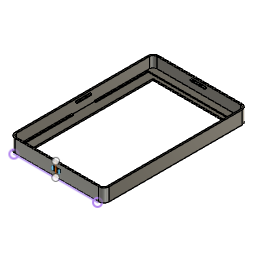
Front+Cover_small (Autodesk Fusion 360 archive; units mm, degrees)
design "Front Cover_small"
Autodesk Fusion 360 part; units mm, degrees
sketch "Outer Dimensions" plane through (0, 0, 0) normal (0, 0, 1) x (1, 0, 0)
  line L0 (117.36, 12) -> (117.36, 183)
  line L1 (125.5, 8.5) -> (125.5, 186.5)
  line L2 (16.04, 178.6) -> (16.04, 16.4)
  line L3 (112.96, 16.4) -> (112.96, 178.6)
  line L4 (3.5, 191.5) -> (125.5, 3.5) construction
  circle A0 centre (8.25, 8.75) radius 1.5
  line L5 (5.36, 12) -> (117.36, 12)
  circle A1 centre (120.75, 8.75) radius 1.5
  circle A2 centre (120.75, 186.25) radius 1.5
  line L6 (8.5, 3.5) -> (120.5, 3.5)
  line L7 (112.96, 178.6) -> (16.04, 16.4) construction
  line L8 (5.36, 82.4713) -> (1.5, 82.4713)
  line L9 (117.36, 183) -> (5.36, 183)
  line L10 (16.04, 16.4) -> (112.96, 16.4)
  line L11 (16.04, 178.6) -> (112.96, 16.4) construction
  line L12 (1.5, 112.5) -> (5.36, 112.5)
  circle A3 centre (8.25, 186.25) radius 1.5
  line L13 (120.5, 191.5) -> (8.5, 191.5)
  line L14 (5.36, 112.5) -> (5.36, 82.4713)
  line L15 (125.5, 191.5) -> (3.5, 3.5) construction
  line L16 (112.96, 178.6) -> (16.04, 178.6)
  line L17 (5.36, 183) -> (5.36, 12)
  line L18 (3.5, 186.5) -> (3.5, 8.5)
  arc A4 (8.5, 191.5) -> (3.5, 186.5) centre (8.5, 186.5) ccw
  arc A5 (3.5, 8.5) -> (8.5, 3.5) centre (8.5, 8.5) ccw
  arc A6 (120.5, 3.5) -> (125.5, 8.5) centre (120.5, 8.5) ccw
  arc A7 (125.5, 186.5) -> (120.5, 191.5) centre (120.5, 186.5) ccw
  line L19 (1.5, 186.5) -> (1.5, 8.5)
  arc A8 (1.5, 8.5) -> (8.5, 1.5) centre (8.5, 8.5) ccw
  line L20 (8.5, 1.5) -> (120.5, 1.5)
  arc A9 (120.5, 1.5) -> (127.5, 8.5) centre (120.5, 8.5) ccw
  line L21 (127.5, 8.5) -> (127.5, 186.5)
  arc A10 (127.5, 186.5) -> (120.5, 193.5) centre (120.5, 186.5) ccw
  line L22 (120.5, 193.5) -> (8.5, 193.5)
  arc A11 (8.5, 193.5) -> (1.5, 186.5) centre (8.5, 186.5) ccw
  point P0 (64.5, 97.5)
  point P1 (8.25, 186.25)
  point P2 (120.75, 8.75)
  point P3 (8.25, 8.75)
  point P4 (120.75, 186.25)
  point P5 (8.25, 8.75)
  point P6 (120.75, 8.75)
  point P7 (64.5, 97.5)
  point P8 (64.5, 97.5)
  point P9 (64.5, 97.5)
  point P10 (64.5, 97.5)
  dimension "d61" = 96.92
  dimension "d62" = 162.2
  dimension "d63" = 112
  dimension "d64" = 171
  dimension "d65" = 4.4
  dimension "d66" = 4.4
  dimension "d84" = 5
  dimension "d88" = 5
  dimension "d90" = 5
  dimension "d98" = 3
  dimension "d102" = 5.25
  dimension "d103" = 4.75
  dimension "d104" = 2
  dimension "d105" = 7
  dimension "d109" = 122
  dimension "d110" = 188
  constraint horizontal L16
  constraint perpendicular L2 L16
  constraint parallel L10 L16
  constraint parallel L2 L3
  constraint coincident P10 L7
  constraint coincident P10 L11
  constraint coincident P10 P9
  constraint horizontal L5
  constraint vertical L0
  constraint horizontal L9
  constraint vertical L17
  constraint horizontal L8
  constraint horizontal L12
  constraint vertical L14
  constraint coincident L8.start L17
  constraint coincident L4.start L18
  constraint coincident L4.start L13
  constraint tangent L18 A4
  constraint tangent L13 A4
  constraint coincident L15.start L13
  constraint coincident L15.start L1
  constraint coincident L15.end L18
  constraint coincident L15.end L6
  constraint tangent L18 A5
  constraint tangent L6 A5
  constraint coincident L4.end L6
  constraint coincident L4.end L1
  constraint tangent L6 A6
  constraint tangent L1 A6
  measures "d61" distance of L2.end L3.start
  measures "d62" distance of L2.start L2.end
  measures "d63" distance of L5.start L0.start
  measures "d64" distance of L9.end L5.start
  measures "d65" distance of L9 L16
  measures "d66" distance of L0 L3
  measures "d84" radius of A4
  measures "d88" radius of A5
  measures "d90" radius of A6
  measures "d98" diameter of A2
  measures "d102" distance of P4 L13
  measures "d103" distance of P4 L1
  measures "d105" radius of A10
  measures "d109" distance of L1 L18
  measures "d110" distance of L6 L13
extrude "Extrude7" add sketch "Outer Dimensions" along normal blind 2 contours L0 L5 L9 L14 L17 | L2 L3 L10 L16 makes body 1
extrude "Extrude9" add sketch "Outer Dimensions" along normal blind 2 contours L8 L12 L14 L17 L18 bodies 1
extrude "Extrude10" add sketch "Outer Dimensions" along normal blind 17.5 contours L1 L6 L8 L12 L13 L18 A4 A5 A6 A7 L19 A8 L20 A9 L21 A10 L22 A11 | L8 L12 L18 L19 bodies 1
extrude "Extrude11" add sketch "Outer Dimensions" along normal blind 3.2 separate body contours A0 | A1 | A2 | A3 makes body 2 at (121.1563, 187.6939, 2.1333) makes body 3 at (9.7425, 8.6006, 2.1333) makes body 4 at (9.0638, 184.99, 2.1333) makes body 5 at (120.2723, 7.3281, 2.1333)
extrude "Extrude14" add sketch "Outer Dimensions" along normal blind 3.2 contours L0 L1 L5 L6 L8 L9 L12 L13 L17 L18 A4 A5 A6 A7 bodies 1 2 3 4 5
extrude "Extrude12" cut sketch "Outer Dimensions" along normal blind 2 contours L2 L3 L10 L16 bodies 1
sketch "Sketch4" plane through (0, 0, 0) normal (0, 1, 0) x (1, 0, 0)
  line L0 (60, -8) -> (69, -8)
  line L1 (69, -8) -> (69, -11.5)
  line L2 (69, -11.5) -> (60, -11.5)
  line L3 (60, -11.5) -> (60, -8)
  line L4 (64.5, -0.8) -> (64.5, -19.8)
  line L5 (64.5, -11.5) -> (64.5, -8)
  line L6 (8.5, 0) -> (120.5, 0)
  dimension "d79" = 3.5
  dimension "d81" = 9
  dimension "d106" = 8
  constraint horizontal L0
  constraint vertical L1
  constraint horizontal L2
  constraint vertical L3
  constraint midpoint L2 L5.start
  constraint midpoint L0 L5.end
  constraint collinear L4 L5
  measures "d79" distance of L0.start L2.end
  measures "d81" distance of L1 L3
  measures "d106" distance of L0 L6
extrude "Extrude13" cut sketch "Sketch4" along normal blind 6 bodies 1
sketch "Skizze5" plane through (3.5, 0, 0) normal (1, 0, 0) x (0, 1, 0)
  line L0 (112.5, 2) -> (112.5, 3.2)
  line L1 (112.5, 3.2) -> (186.5, 3.2)
  line L2 (186.5, 3.2) -> (186.5, 17.5)
  line L3 (186.5, 17.5) -> (8.5, 17.5)
  line L4 (8.5, 17.5) -> (8.5, 3.2)
  line L5 (82.4713, 3.2) -> (82.4713, 2)
  line L6 (82.4713, 2) -> (112.5, 2)
  line L7 (107.5, 15) -> (87.5, 15)
  line L8 (87.5, 15) -> (87.5, 13)
  line L9 (87.5, 13) -> (107.5, 13)
  line L10 (107.5, 13) -> (107.5, 15)
  line L11 (107.5, 15) -> (87.5, 13) construction
  line L12 (87.5, 15) -> (107.5, 13) construction
  line L13 (97.5, 14) -> (97.5, 17.5)
  line L14 (8.5, 3.2) -> (82.4713, 3.2)
  point P0 (97.5, 14)
  point P1 (97.5, 14)
  dimension "d111" = 20
  dimension "d112" = 2
  dimension "d127" = 3.5
  constraint horizontal L7
  constraint perpendicular L7 L8
  constraint parallel L7 L9
  constraint parallel L8 L10
  constraint coincident L11 P1
  constraint coincident L12 P1
  constraint coincident P1 P0
  constraint midpoint L3 L13.end
  measures "d111" distance of L8.end L9.end
  measures "d112" distance of L7.end L8.end
  measures "d127" distance of P1 L13.end
extrude "Extrusion15" add sketch "Skizze5" along normal blind 2 contours L7 L8 L9 L10 bodies 1
chamfer "Fase1" distance 0.5 distance2 1.5 4 edges at (5.5, 97.5, 15) (5.5, 87.5, 14) (5.5, 97.5, 13) (5.5, 107.5, 14) measured on face at (5.5, 94.1667, 14.3333) measured on face at (5.5, 94.1667, 14.3333) measured on face at (5.5, 94.1667, 14.3333) measured on face at (5.5, 94.1667, 14.3333) on bodies 1
sketch "Skizze6" plane through (125.5, 0, 0) normal (-1, 0, 0) x (0, -1, 0)
  line L0 (-186.5, 3.2) -> (-8.5, 3.2)
  line L1 (-8.5, 3.2) -> (-8.5, 17.5)
  line L2 (-8.5, 17.5) -> (-186.5, 17.5)
  line L3 (-186.5, 17.5) -> (-186.5, 3.2)
  line L4 (-87.5, 15) -> (-107.5, 15)
  line L5 (-87.5, 13) -> (-87.5, 15)
  line L6 (-107.5, 15) -> (-107.5, 13)
  line L7 (-107.5, 13) -> (-87.5, 13)
extrude "Extrusion16" add sketch "Skizze6" along normal blind 2 contours L4 L5 L6 L7 bodies 1
chamfer "Fase2" distance 0.5 distance2 1.5 4 edges at (123.5, 97.5, 15) (123.5, 107.5, 14) (123.5, 97.5, 13) (123.5, 87.5, 14) measured on face at (123.5, 100.8333, 14.3333) measured on face at (123.5, 100.8333, 14.3333) measured on face at (123.5, 100.8333, 14.3333) measured on face at (123.5, 100.8333, 14.3333) on bodies 1
sketch "Skizze7" plane through (0, 191.5, 0) normal (0, -1, 0) x (1, 0, 0)
  line L0 (8.5, 3.2) -> (120.5, 3.2)
  line L1 (120.5, 3.2) -> (120.5, 17.5)
  line L2 (120.5, 17.5) -> (8.5, 17.5)
  line L3 (8.5, 17.5) -> (8.5, 3.2)
  line L4 (64.5, 14) -> (64.5, 17.5)
  line L5 (54.5, 13) -> (74.5, 13)
  line L6 (74.5, 13) -> (74.5, 15)
  line L7 (74.5, 15) -> (54.5, 15)
  line L8 (54.5, 15) -> (54.5, 13)
  line L9 (54.5, 13) -> (74.5, 15) construction
  line L10 (74.5, 13) -> (54.5, 15) construction
  point P0 (64.5, 14)
  point P1 (64.5, 14)
  point P2 (64.5, 14)
  dimension "d128" = 3.5
  dimension "d129" = 20
  dimension "d130" = 2
  constraint coincident P2 P1
  constraint midpoint L2 L4.end
  constraint perpendicular L2 L4
  constraint horizontal L5
  constraint perpendicular L5 L6
  constraint parallel L5 L7
  constraint parallel L6 L8
  constraint coincident L9 P2
  constraint coincident L10 P2
  measures "d128" distance of P2 L4.end
  measures "d129" distance of L6.end L7.end
  measures "d130" distance of L5.end L6.end
extrude "Extrusion17" add sketch "Skizze7" along normal blind 2 contours L5 L6 L7 L8 bodies 1
chamfer "Fase3" distance 0.5 distance2 1.5 4 edges at (64.5, 189.5, 15) (74.5, 189.5, 14) (64.5, 189.5, 13) (54.5, 189.5, 14) measured on face at (61.1667, 189.5, 14.3333) measured on face at (61.1667, 189.5, 14.3333) measured on face at (61.1667, 189.5, 14.3333) measured on face at (61.1667, 189.5, 14.3333) on bodies 1
sketch "Skizze9" plane through (0, 3.5, 0) normal (0, 1, 0) x (-1, 0, 0)
  line L0 (-60, 11.5) -> (-60, 8)
  line L1 (-60, 8) -> (-69, 8)
  line L2 (-69, 8) -> (-69, 11.5)
  line L3 (-69, 11.5) -> (-60, 11.5)
  line L4 (-120.5, 3.2) -> (-8.5, 3.2)
  line L5 (-8.5, 3.2) -> (-8.5, 17.5)
  line L6 (-8.5, 17.5) -> (-120.5, 17.5)
  line L7 (-120.5, 17.5) -> (-120.5, 3.2)
  line L8 (-54.5, 15) -> (-74.5, 15)
  line L9 (-54.5, 13) -> (-54.5, 15)
  line L10 (-74.5, 13) -> (-54.5, 13)
  line L11 (-74.5, 15) -> (-74.5, 13)
extrude "Extrusion18" add sketch "Skizze9" along normal blind 2 contours L8 L9 L10 L11 bodies 1
chamfer "Fase4" distance 0.5 distance2 1.5 4 edges at (64.5, 5.5, 15) (54.5, 5.5, 14) (64.5, 5.5, 13) (74.5, 5.5, 14) measured on face at (67.8333, 5.5, 14.3333) measured on face at (67.8333, 5.5, 14.3333) measured on face at (67.8333, 5.5, 14.3333) measured on face at (67.8333, 5.5, 14.3333) on bodies 1
equation "d61 = 97.92 mm - 1 mm"
equation "d62 = 163.2 mm - 1 mm"
equation "d63 = 111.2 mm + 0.8 mm"
equation "d64 = 170.2 mm + 0.8 mm"
